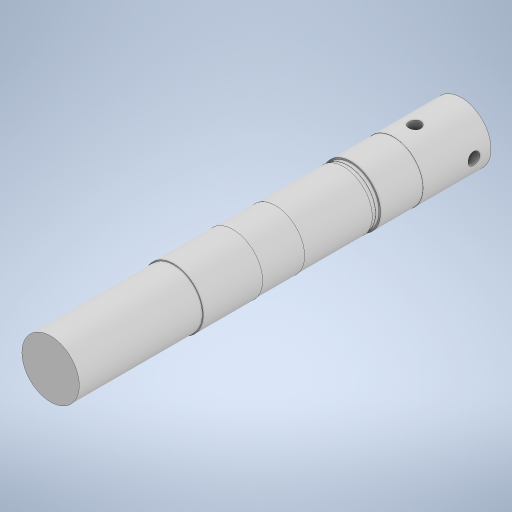
# Autodesk Inventor part: Mangon_Conduccion
Saved by Autodesk Inventor 2024 (Build 280153000, 153)
## iProperties
Created: 2026-01-05
Part Number: Mangon_Conduccion
Material: Generic
Document SubType Name: Modeling
Designer: eduso
Density: 1 g/cm^3
Appearance: Default
Testero_007: 4.000 mm
Espacio_008: 50,000 mm
Inteerior_Tubo_009: 80,000 mm
Author: eduso
Autodesk Inventor part; units mm, degrees
ref_plane "YZ Plane" through (0, 0, 0) normal (1, 0, 0) x (0, 1, 0)
ref_plane "XY Plane" through (0, 0, 0) normal (0, 0, 1) x (1, 0, 0)
sketch "Sketch1" plane through (0, 0, 0) normal (0, 1, 0) x (-1, 0, 0)
  line L0 (32.75, 5) -> (33.95, 5)
  line L1 (33.95, 5) -> (33.95, 85)
  line L2 (33.95, 85) -> (34.25, 85)
  line L3 (34.25, 85) -> (34.25, 135)
  line L4 (34.25, 135) -> (34.75, 135)
  line L5 (34.75, 135) -> (34.75, 205)
  line L6 (34.75, 205) -> (33.75, 205)
  line L7 (33.75, 205) -> (33.75, 245)
  line L8 (33.75, 245) -> (33.75, 245)
  line L9 (33.75, 245) -> (33.75, 350)
  line L10 (33.75, 350) -> (0, 350)
  line L11 (0, 189.8856) -> (0, -122.7414) construction
  line L12 (32.75, 5) -> (32.75, 0)
  line L13 (0, 350) -> (0, 0)
  line L14 (32.75, 0) -> (32.95, 0)
  line L15 (32.95, 0) -> (32.95, -4)
  line L16 (32.95, -4) -> (34.65, -4)
  line L17 (34.65, -4) -> (34.65, -54)
  line L18 (34.65, -54) -> (34.85, -54)
  line L19 (34.85, -54) -> (34.85, -134)
  line L20 (34.85, -134) -> (0, -134)
  line L21 (0, 0) -> (0, -134)
  line L22 (32.75, 0) -> (32.95, 0)
  dimension "d0" = 105
  dimension "d3" = 70
  dimension "d2" = 80
  dimension "d4" = 5
  dimension "d15" = 40
  dimension "d16" = 50
  dimension "d69" = 33.75
  dimension "d70" = 34.75
  dimension "d71" = 33.95
  dimension "d78" = 32.75
  dimension "d82" = 4
  dimension "d83" = 50
  dimension "d84" = 32.95
  dimension "d85" = 34.85
  dimension "d86" = 80
  dimension "d87" = 33.75
  dimension "d88" = 34.25
  dimension "d89" = 34.65
  constraints: 46 end point, 10 perpendicular, 3 horizontal, 3 vertical, 2 collinear, 1 point on line, 3 other
  measures "d0" distance of L8.end L9.end
  measures "d3" distance of L4.end L5.end
  measures "d2" distance of L0.end L1.end
  measures "d4" distance of L0.start L12.end
  measures "d15" distance of L6.end L7.end
  measures "d16" distance of L2.end L3.end
  measures "d69" distance between parallel lines of L13 L9
  measures "d70" distance between parallel lines of L13 L5
  measures "d71" distance between parallel lines of L1 L13
  measures "d78" distance between parallel lines of L11 L12
  measures "d82" distance of L14.end L15.end
  measures "d83" distance of L16.end L17.end
  measures "d84" distance between parallel lines of L11 L15
  measures "d85" distance between parallel lines of L21 L19
  measures "d86" distance of L18.end L19.end
  measures "d87" distance between parallel lines of L13 L7
  measures "d88" distance between parallel lines of L11 L3
  measures "d89" distance between parallel lines of L11 L17
ref_plane "Work Plane1" through (0, 15, 0) normal (0, 1, 0) x (-1, 0, 0)
sketch "Sketch2" plane through (0, 15, 0) normal (0, 1, 0) x (-1, 0, 0)
  arc A0 (-5, 259) -> (5, 259) centre (0, 259) ccw
  arc A1 (5, 334) -> (-5, 334) centre (0, 334) ccw
  line L0 (-5, 334) -> (-5, 259)
  line L1 (5, 334) -> (5, 259)
  line L2 (0, 0) -> (0, 401.4271) construction
  dimension "d18" = 10
  dimension "d19" = 10
  dimension "d65" = 259
  dimension "d68" = 75
  constraints: 6 end point, 4 point on circle, 3 tangent, 2 centre point, 2 point on line, 1 parallel, 1 vertical
  measures "d18" diameter of A0
  measures "d19" diameter of A1
  measures "d65" distance of L2.start A0.centre
  measures "d68" distance of A1.centre A0.centre
sketch "Sketch3" plane through (0, 15, 0) normal (0, 1, 0) x (-1, 0, 0)
  circle A0 centre (0, -79) radius 7
  point P0 (0, 0)
  dimension "d22" = 14
  dimension "d66" = 79
  constraints: 1 centre point
  measures "d22" diameter of A0
  measures "d66" distance of point (0, 0) A0.centre
sketch "Sketch4" plane through (0, 0, 0) normal (1, 0, 0) x (0, 1, 0)
  circle A0 centre (0, -114) radius 7
  point P0 (0, 0)
  dimension "d28" = 14
  dimension "d67" = 114
  constraints: 1 centre point
  measures "d28" diameter of A0
  measures "d67" distance of point (0, 0) A0.centre
revolve "Revolution1" add sketch "Sketch1" angle 360 about axis through (0, 0, 350) along (0, 0, -1)
extrude "Extrusion4" cut sketch "Sketch2" along normal blind 10
extrude "Extrusion5" cut sketch "Sketch3" along normal blind 20 and the other way blind 45
extrude "Extrusion6" cut sketch "Sketch4" along normal blind 35 and the other way blind 30
sketch "Sketch5" plane through (0, 0, 0) normal (0, 1, 0) x (-1, 0, 0)
  line L0 (32.75, 5) -> (32.75, 0) projected
  point P0 (0, 0)
sketch "Sketch6" plane through (0, 0, 0) normal (1, 0, 0) x (0, 1, 0)
  line L0 (0, 0) -> (-46.2751, 0) construction
  constraints: 2 end point, 1 horizontal
equation "\"espesor_testero\" = 4"
equation "\"espesor_brida\" = 5"
body "Solid4"
